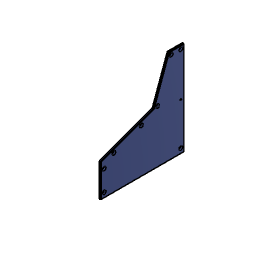
Panneau latéral droit (Autodesk Fusion 360 design; units mm, degrees)
Autodesk Fusion 360 part; units mm, degrees
note: some values were not read from the file. Chosen so that the rebuilt part matches the saved one: which face or edge a step refers to. Set by a fixed rule: which sketch regions a step uses.
sketch "Sketch1" plane through (71.9136, 0, 0) normal (1, 0, 0) x (0, 0, -1)
  line L0 (-131.1911, 0) -> (-128.1911, 0)
  line L1 (-128.1911, 0) -> (-128.1911, 63)
  line L2 (-128.1911, 63) -> (-131.1911, 63)
  line L3 (-131.1911, 63) -> (-131.1911, 0)
  line L4 (-128.1911, 0) -> (30.8089, 0)
  line L5 (30.8089, 0) -> (30.8089, 178.9785)
  line L6 (1.6489, 178.9785) -> (-27.1828, 99.764)
  line L7 (-27.1828, 99.764) -> (-128.1911, 63)
  line L8 (-128.1911, 63) -> (-128.1911, 0)
  line L9 (30.8089, 0) -> (-128.1911, 0)
  line L10 (1.6489, 178.9785) -> (30.8089, 178.9785)
  line L11 (33.8089, 178.9785) -> (1.6489, 178.9785)
  circle A0 centre (-121.8411, 9.35) radius 1.5
  circle A1 centre (-121.8411, 48.35) radius 1.25
  circle A2 centre (-103.3298, 65.2912) radius 1.25
  circle A3 centre (-50.9889, 84.3418) radius 1.25
  circle A4 centre (6.0952, 172.6285) radius 1.25
  circle A5 centre (-121.8411, 48.35) radius 1.5
  circle A6 centre (-103.3298, 65.2912) radius 1.5
  circle A7 centre (-50.9889, 84.3418) radius 1.5
  circle A8 centre (-19.9674, 101.0221) radius 1.5
  circle A9 centre (6.0952, 172.6285) radius 1.5
  line L12 (30.8089, 185.0295) -> (30.8089, 177.2256) construction
  line L13 (33.8089, 181.9785) -> (33.8089, 178.9785) construction
  circle A10 centre (24.4589, 172.6285) radius 1.5
  circle A11 centre (24.4589, 9.35) radius 1.5
  circle A12 centre (24.2089, 89.4893) radius 1.5
  point P0 (2.7408, 181.9785)
  point P1 (-27.1828, 99.764)
  dimension "d241" = 3
  dimension "d242" = 3
  dimension "d243" = 3
  dimension "d244" = 3
  dimension "d245" = 3
  dimension "d277" = 3
  dimension "d331" = 3
  constraint coincident L0.end L1.start
  constraint perpendicular L1 L4
  constraint equal L1 L8
  constraint parallel L1 L8
  constraint equal L4 L9
  constraint coincident L11.start L13.end
  constraint coincident L6.start L10.start
  constraint concentric A1 A5
  constraint concentric A2 A6
  constraint concentric A3 A7
  constraint concentric A4 A9
  constraint perpendicular L10 L12
  constraint coincident L11 L5.end
  constraint coincident L12 L5.end
  measures "d241" diameter of A5
  measures "d242" diameter of A6
  measures "d243" diameter of A7
  measures "d244" diameter of A8
  measures "d245" diameter of A9
  measures "d277" distance of L12 L13
  measures "d331" diameter of A12
extrude "Extrude1" add sketch "Sketch1" against normal blind 3 contours L1 L4 L5 L6 L7 L8 L9 L10 L11 makes body 1
chamfer "Chamfer2" distance 2 angle 45 8 edges at (71.9136, 9.35, 123.3411) (71.9136, 48.35, 123.3411) (71.9136, 65.2912, 104.8298) (71.9136, 84.3418, 52.4889) (71.9136, 9.35, -22.9589) (71.9136, 101.0221, 21.4674) (71.9136, 172.6285, -4.5952) (71.9136, 172.6285, -22.9589) on bodies 1
mirror "Mirror1" about plane through (14.9136, 89.4893, -32.3089) normal (1, 0, 0) of bodies 1 makes body 2
copy_body "Body->Comp1" bodies 2 removing the originals makes body 3 in component "Panneau latéral gauche"
chamfer "Chamfer3" distance 0.6 angle 45 6 edges at (71.9136, 31.5, 128.1911) (71.9136, 81.382, 77.687) (71.9136, 139.3713, 12.7669) (71.9136, 178.9785, -16.2289) (71.9136, 89.4893, -30.8089) (71.9136, 0, 48.6911) on bodies 1
equation "d238 = -EpaisseurParoi"
equation "d277 = EpaisseurParoi"
equation "EpaisseurParoi = 3 mm"
